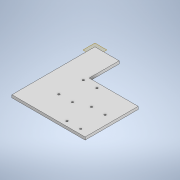
# Autodesk Inventor part: borard2_L
Saved by Autodesk Inventor 2020 (Build 240168000, 168)
## iProperties
Created: 2022-07-25
Part Number: borard2_L
Material: 일반
Document SubType Name: Modeling
Designer: SeungJin
Density: 1 g/cm^3
Appearance: 기본값
Author: SeungJin
Autodesk Inventor part; units mm, degrees
ref_plane "YZ Plane" through (0, 0, 0) normal (1, 0, 0) x (0, 1, 0)
ref_plane "XZ Plane" through (0, 0, 0) normal (0, 1, 0) x (-1, 0, 0)
ref_plane "XY Plane" through (0, 0, 0) normal (0, 0, 1) x (1, 0, 0)
ref_plane "작업 평면1" through (-145.5, 0, 75) normal (0, 1, 0) x (1, 0, 0)
sketch "스케치1" plane through (-145.5, 0, 75) normal (0, 1, 0) x (1, 0, 0)
  line L0 (0, -152.5) -> (185.5, -152.5)
  line L1 (185.5, -152.5) -> (185.5, 10)
  line L2 (185.5, 10) -> (75, 10)
  line L3 (75, 10) -> (75, 0)
  line L4 (75, 0) -> (0, 0)
  line L5 (0, 0) -> (0, -152.5)
  line L6 (185.5, 10) -> (75, 10)
  line L7 (185.5, 10) -> (34.5, 10)
  line L8 (34.5, 10) -> (34.5, -55)
  line L9 (34.5, -55) -> (185.5, -55)
  line L10 (185.5, -55) -> (185.5, 10)
  line L11 (44.5, -55) -> (44.5, 10)
  line L12 (195.5, 10) -> (195.5, -55)
  line L13 (134.5, -152.5) -> (134.5, -55)
  point P0 (44.5, 0)
  dimension "d1" = 151
  dimension "d2" = 65
  dimension "d3" = 10
  dimension "d4" = 10
  dimension "d27" = 90
  constraints: 28 end point, 4 point on line, 1 perpendicular, 1 other
  measures "d1" distance of L9.end L8.end
  measures "d2" distance of L8.end L7.end
  measures "d3" distance between parallel lines of L11 L8
  measures "d4" distance between parallel lines of L12 L1
  measures "d27" distance between parallel lines of L13 L11
extrude "돌출1" add sketch "스케치1" along normal blind 5 contours L5 L4 L8 L9 L13 L0 | L4 L11 L9 L8
sketch "스케치3" plane through (-145.5, 0, 75) normal (0, -1, 0) x (1, 0, 0)
  line L0 (44.5, 55) -> (44.5, 0) projected
  line L1 (134.5, 55) -> (44.5, 55) projected
  line L2 (0, 152.5) -> (134.5, 152.5) projected
  line L3 (0, 0) -> (0, 152.5) projected
  line L4 (44.5, 0) -> (0, 0) projected
  line L5 (30, 146.25) -> (130, 146.25)
  line L6 (130, 146.25) -> (130, 61.25)
  line L7 (130, 61.25) -> (30, 61.25)
  line L8 (30, 61.25) -> (30, 146.25)
  line L9 (130, 146.25) -> (80, 146.25)
  line L10 (80, 146.25) -> (80, 96.25)
  line L11 (80, 96.25) -> (130, 96.25)
  line L12 (130, 96.25) -> (130, 146.25)
  line L13 (30, 61.25) -> (80, 61.25)
  line L14 (80, 61.25) -> (80, 111.25)
  line L15 (80, 111.25) -> (30, 111.25)
  line L16 (30, 111.25) -> (30, 61.25)
  line L17 (117.5, 143.75) -> (92.5, 143.75)
  line L18 (92.5, 143.75) -> (92.5, 98.75)
  line L19 (92.5, 98.75) -> (117.5, 98.75)
  line L20 (117.5, 98.75) -> (117.5, 143.75)
  line L21 (67.5, 108.75) -> (42.5, 108.75)
  line L22 (42.5, 108.75) -> (42.5, 63.75)
  line L23 (42.5, 63.75) -> (67.5, 63.75)
  line L24 (67.5, 63.75) -> (67.5, 108.75)
  line L25 (44.5, 0) -> (0, 0) projected
  line L26 (134.5, 152.5) -> (134.5, 55) projected
  point P0 (145.5, -75)
  point P1 (130, 103.75)
  point P2 (30, 103.75)
  point P3 (117.5, 121.25)
  point P4 (130, 121.25)
  point P5 (105, 143.75)
  point P6 (105, 146.25)
  point P7 (67.5, 86.25)
  point P8 (80, 86.25)
  point P9 (55, 108.75)
  point P10 (55, 111.25)
  dimension "d9" = 100
  dimension "d10" = 85
  dimension "d11" = 50
  dimension "d12" = 50
  dimension "d13" = 50
  dimension "d14" = 25
  dimension "d15" = 45
  dimension "d16" = 25
  dimension "d17" = 45
  dimension "d26" = 30
  constraints: 40 end point, 10 midpoint, 8 coincident, 2 vertical alignment, 1 point on line
  measures "d9" distance of L6.end L7.end
  measures "d10" distance of L5.end L6.end
  measures "d11" distance of L11.end L10.end
  measures "d12" distance of L10.end L9.end
  measures "d13" distance of L14.end L13.end
  measures "d14" distance of L19.end L18.end
  measures "d15" distance of L18.end L17.end
  measures "d16" distance of L23.end L22.end
  measures "d17" distance of L22.end L21.end
  measures "d26" distance between parallel lines of L3 L8
hole "구멍1" at (-28, 0, 218.75) at (-28, 0, 173.75) at (-53, 0, 218.75) at (-53, 0, 173.75) at (-78, 0, 183.75) at (-103, 0, 183.75) at (-103, 0, 138.75) at (-78, 0, 138.75) direction (0, 1, 0) diameter 3.4 end through all counterbore diameter 6 counterbore depth 3 clearance for "Hex Head Cap Screw ISO 24017" size "M3" standard "ISO"
